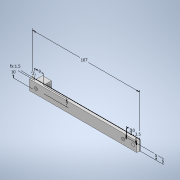
# Autodesk Inventor part: button_bar
Saved by Autodesk Inventor 2020 (Build 240168000, 168)
## iProperties
Created: 2022-09-30
Part Number: button_bar
Material: 일반
Document SubType Name: Modeling
Designer: taewo
Density: 1 g/cm^3
Appearance: 기본값
Author: taewo
Autodesk Inventor part; units mm, degrees
ref_plane "YZ Plane" through (0, 0, 0) normal (1, 0, 0) x (0, 1, 0)
ref_plane "XZ Plane" through (0, 0, 0) normal (0, 1, 0) x (-1, 0, 0)
ref_plane "XY Plane" through (0, 0, 0) normal (0, 0, 1) x (1, 0, 0)
sketch "sketch" plane through (0, 0, 0) normal (0, 0, 1) x (1, 0, 0)
  line L0 (-21.4, 0) -> (128.4, 0) construction
  line L1 (0, -2) -> (0, 12) construction
  line L2 (0, 10) -> (107, 10)
  line L3 (107, 10) -> (107, 0)
  line L4 (107, 0) -> (0, 0)
  line L5 (0, 0) -> (0, 10)
  line L6 (2, 8.5) -> (11, 8.5)
  line L7 (11, 8.5) -> (11, 1.5)
  line L8 (11, 1.5) -> (2, 1.5)
  line L9 (2, 1.5) -> (2, 8.5)
  circle A0 centre (93.5, 5) radius 1.5
  circle A1 centre (103.5, 5) radius 1.5
  dimension "d0" = 10
  dimension "d1" = 107
  dimension "d2" = 9
  dimension "d3" = 7
  dimension "d4" = 1.5
  dimension "d5" = 2
  dimension "d6" = 3
  dimension "d7" = 3
  dimension "d8" = 3.5
  dimension "d9" = 10
  dimension "d10" = 5
  dimension "d11" = 5
  constraints: 16 end point, 4 parallel, 2 centre point, 2 horizontal, 2 perpendicular
  measures "d0" distance of L4.end L2.start
  measures "d1" distance of L2.start L2.end
  measures "d2" distance of L6.start L6.end
  measures "d3" distance of L6.end L7.end
  measures "d4" distance between parallel lines of L2 L6
  measures "d5" distance between parallel lines of L1 L9
  measures "d6" diameter of A0
  measures "d7" diameter of A1
  measures "d8" distance from line of L3 A1.centre
  measures "d9" distance of A1.centre A0.centre
  measures "d10" distance from line of L4 A0.centre
  measures "d11" distance from line of L4 A1.centre
extrude "body" add sketch "sketch" along normal blind 3 contours L2 L3 L4 L5 | L6 L7 L8 L9
extrude "button" add sketch "sketch" against normal blind 8 contours L6 L7 L8 L9
sketch "button_sketch" plane through (0, 0, 3) normal (0, 0, 1) x (1, 0, 0)
  line L0 (11, 1.5) -> (2, 1.5) projected
  line L1 (11, 8.5) -> (2, 8.5) projected
  line L2 (2, 8.5) -> (2, 1.5) projected
  line L3 (11, 1.5) -> (11, 8.5) projected
  circle A0 centre (6.5, 5) radius 1.5
  line L4 (107, 10) -> (0, 10) projected
  point P0 (0, 0)
  dimension "d16" = 3
  dimension "d17" = 5
  dimension "d18" = 4.5
  constraints: 1 centre point
  measures "d16" diameter of A0
  measures "d17" distance from line of L4 A0.centre
  measures "d18" distance from line of L2 A0.centre
extrude "bolt" cut sketch "button_sketch" against normal blind 8 contours A0
equation "\"d4\" = -0.5 * d3 + 0.5 * d0"
equation "\"d17\" = 0.5 * d0"
equation "\"d18\" = 0.5 * d2"
